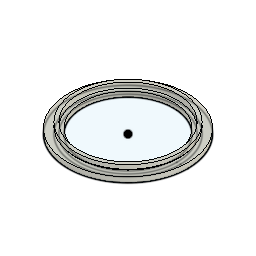
Bottom Teflon Ring v1 (Autodesk Fusion 360 design; units mm, degrees)
Autodesk Fusion 360 part; units mm, degrees
sketch "Sketch1" plane through (0, 0, 0) normal (0, 0, 1) x (1, 0, 0)
  circle A0 centre (0, 0) radius 67.4
  circle A1 centre (0, 0) radius 89
  circle A2 centre (0, 0) radius 72.8
  circle A3 centre (0, 0) radius 78.05
  dimension "d1" = 134.8
  dimension "d2" = 178
  dimension "d3" = 145.6
  dimension "d4" = 156.1
  constraint coincident A0.centre A1.centre
  constraint concentric A0 A1
  measures "d1" diameter of A0
  measures "d2" diameter of A1
  measures "d3" diameter of A2
  measures "d4" diameter of A3
extrude "Extrude1" add sketch "Sketch1" along normal blind 7.7 contours A1 makes body 1
extrude "Extrude2" add sketch "Sketch1" along normal blind 7.7 separate body contours A2 makes body 2
extrude "Extrude4" add sketch "Sketch1" along normal blind 15.6 contours A3 bodies 1 2
sketch "Sketch3" plane through (0, 0, 7.7) normal (0, 0, 1) x (-1, 0, 0)
  circle A0 centre (0, 0) radius 78.05
  circle A1 centre (0, 0) radius 89
  circle A2 centre (0, 0) radius 76.55
  circle A3 centre (0, 0) radius 77.8
  dimension "d13" = 153.1
  constraint coincident A0.centre A1.centre
  constraint concentric A2 A3
  measures "d13" diameter of A2
extrude "Extrude5" cut sketch "Sketch3" along normal blind 2 contours A0 | A3 bodies 1
extrude "Extrude3" [suppressed]
equation "d2 = 135 mm + ( 21.8 * 2 ) * 1 mm - 0.6 mm"
equation "d4 = 145.600 mm + 10.5 mm"
equation "d13 = 155.600 mm - 2.5 mm"
